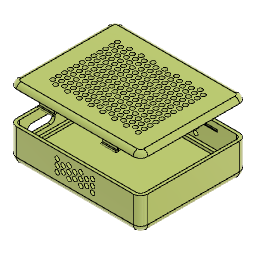
esp32_mesh_node (Autodesk Fusion 360 design; units mm, degrees)
Autodesk Fusion 360 part; units mm, degrees
note: some values were not read from the file. Set by a fixed rule: which sketch regions a step uses.
sketch "Sketch1" plane through (0, 0, 0) normal (0, 0, 1) x (1, 0, 0)
  line L0 (0, 0) -> (44.5, 0)
  line L1 (44.5, 0) -> (44.5, 36)
  line L2 (44.5, 36) -> (0, 36)
  line L3 (0, 36) -> (0, 0)
  dimension "d1" = 44.5
  dimension "d2" = 36
  constraint horizontal L0
  constraint vertical L1
  constraint horizontal L2
  constraint vertical L3
  constraint coincident L0.start L3.end
  measures "d1" distance of L0.start L0.end
  measures "d2" distance of L0.start L2.end
extrude "Extrude1" add sketch "Sketch1" along normal blind 2.5 makes body 1
sketch "Sketch2" plane through (0, 0, 2.5) normal (0, 0, 1) x (-1, 0, 0)
  line L0 (0, -36) -> (0, 0)
  line L1 (0, 0) -> (-44.5, 0)
  line L2 (-44.5, 0) -> (-44.5, -36)
  line L3 (-44.5, -36) -> (0, -36)
  line L4 (-2, -2) -> (-42.5, -2)
  line L5 (-42.5, -2) -> (-42.5, -34)
  line L6 (-42.5, -34) -> (-2, -34)
  line L7 (-2, -34) -> (-2, -2)
  dimension "d5" = -2
extrude "Extrude2" add sketch "Sketch2" along normal blind 8 bodies 1
sketch "Sketch3" plane through (0, 0, 2.5) normal (0, 0, 1) x (-1, 0, 0)
  line L0 (-2, -2) -> (-42.5, -2)
  line L1 (-42.5, -2) -> (-42.5, -34)
  line L2 (-42.5, -34) -> (-2, -34)
  line L3 (-2, -34) -> (-2, -2)
  line L4 (-3.25, -32.75) -> (-41.25, -32.75)
  line L5 (-41.25, -32.75) -> (-41.25, -3.25)
  line L6 (-41.25, -3.25) -> (-3.25, -3.25)
  line L7 (-3.25, -3.25) -> (-3.25, -32.75)
  line L8 (0, -36) -> (0, 0)
  circle A0 centre (-3.25, -32.75) radius 2
  circle A1 centre (-41.25, -32.75) radius 2
  circle A2 centre (-41.25, -3.25) radius 2
  circle A3 centre (-3.25, -3.25) radius 2
  dimension "d18" = 38
  dimension "d20" = 32
  dimension "d21" = 1.25
  dimension "d23" = 40.5
  dimension "d25" = 36
  dimension "d26" = 29.5
  dimension "d27" = 1.25
  dimension "d28" = 4
  dimension "d29" = 4
  dimension "d30" = 4
  dimension "d31" = 4
  constraint horizontal L4
  constraint vertical L5
  constraint horizontal L6
  constraint vertical L7
  constraint coincident L4.start L7.end
  constraint coincident L4.end L5.start
  constraint coincident L5.end L6.start
  constraint coincident L6.end L7.start
  measures "d18" distance of L4.start L4.end
  measures "d20" distance of L0 L2
  measures "d21" distance of L2 L4
  measures "d23" distance of L1 L3
  measures "d25" distance of L8.start L8.end
  measures "d26" distance of L4 L6
  measures "d27" distance of L3 L7
  measures "d28" diameter of A0
  measures "d29" diameter of A1
  measures "d30" diameter of A2
  measures "d31" diameter of A3
extrude "Extrude3" add sketch "Sketch3" along normal blind 1 contours L0 L3 L6 L7 A3 | L0 L1 L5 L6 A2 | L6 L7 A3 | L2 L3 L4 L7 A0 | L5 L6 A2 | L4 L7 A0 | L1 L2 L4 L5 A1 | L4 L5 A1 bodies 1
sketch "Sketch4" plane through (0, 0, 3.5) normal (0, 0, 1) x (-1, 0, 0)
  line L0 (-2, -34) -> (-2, -31.1888)
  arc A0 (-2, -31.1888) -> (-4.8112, -34) centre (-3.25, -32.75) ccw
  line L1 (-4.8112, -34) -> (-2, -34)
  circle A1 centre (-3.25, -32.75) radius 0.9
  line L2 (-2, -2) -> (-4.8112, -2)
  arc A2 (-4.8112, -2) -> (-2, -4.8112) centre (-3.25, -3.25) ccw
  line L3 (-2, -4.8112) -> (-2, -2)
  arc A3 (-42.5, -4.8112) -> (-39.6888, -2) centre (-41.25, -3.25) ccw
  line L4 (-39.6888, -2) -> (-42.5, -2)
  line L5 (-42.5, -2) -> (-42.5, -4.8112)
  arc A4 (-39.6888, -34) -> (-42.5, -31.1888) centre (-41.25, -32.75) ccw
  line L6 (-42.5, -31.1888) -> (-42.5, -34)
  line L7 (-42.5, -34) -> (-39.6888, -34)
  circle A5 centre (-41.25, -32.75) radius 0.9
  circle A6 centre (-41.25, -3.25) radius 0.9
  circle A7 centre (-3.25, -3.25) radius 0.9
  dimension "d34" = 1.8
  dimension "d35" = 1.8
  dimension "d36" = 1.8
  dimension "d37" = 1.8
  constraint concentric A0 A1
  constraint concentric A4 A5
  constraint concentric A3 A6
  constraint concentric A2 A7
  measures "d34" diameter of A1
  measures "d35" diameter of A5
  measures "d36" diameter of A6
  measures "d37" diameter of A7
extrude "Extrude4" add sketch "Sketch4" along normal blind 3 contours A1 | A5 | A6 | A7 bodies 1
sketch "Sketch5" plane through (0, 0, 10.5) normal (0, 0, 1) x (-1, 0, 0)
  line L0 (-2, -2) -> (-2, -34)
  line L1 (-2, -34) -> (-42.5, -34)
  line L2 (-42.5, -34) -> (-42.5, -2)
  line L3 (-42.5, -2) -> (-2, -2)
  line L4 (-44.5, -36) -> (0, -36)
  line L5 (0, -36) -> (0, 0)
  line L6 (0, 0) -> (-44.5, 0)
  line L7 (-44.5, 0) -> (-44.5, -36)
  line L8 (-43.5, -1) -> (-1, -1)
  line L9 (-1, -1) -> (-1, -35)
  line L10 (-1, -35) -> (-43.5, -35)
  line L11 (-43.5, -35) -> (-43.5, -1)
  dimension "d40" = -1
extrude "Extrude5" cut sketch "Sketch5" against normal up to surface (7 mm away) contours L8 L9 L10 L11 bodies 1
sketch "Sketch7" plane through (0, 0, 6.5) normal (0, 0, 1) x (-1, 0, 0)
  circle A0 centre (-3.25, -32.75) radius 1.05
  line L0 (-1, -35) -> (-1, -1)
  line L1 (-1, -1) -> (-43.5, -1)
  line L2 (-43.5, -1) -> (-43.5, -35)
  line L3 (-43.5, -35) -> (-1, -35)
  arc A1 (-42.5, -4.8112) -> (-39.6888, -2) centre (-41.25, -3.25) ccw
  line L4 (-39.6888, -2) -> (-4.8112, -2)
  arc A2 (-4.8112, -2) -> (-2, -4.8112) centre (-3.25, -3.25) ccw
  line L5 (-2, -4.8112) -> (-2, -31.1888)
  arc A3 (-2, -31.1888) -> (-4.8112, -34) centre (-3.25, -32.75) ccw
  line L6 (-4.8112, -34) -> (-39.6888, -34)
  arc A4 (-39.6888, -34) -> (-42.5, -31.1888) centre (-41.25, -32.75) ccw
  line L7 (-42.5, -31.1888) -> (-42.5, -4.8112)
  circle A5 centre (-41.25, -32.75) radius 1.05
  circle A6 centre (-41.25, -3.25) radius 1.05
  circle A7 centre (-3.25, -3.25) radius 1.05
  circle A8 centre (-3.25, -32.75) radius 0.9
  circle A9 centre (-41.25, -32.75) radius 0.9
  circle A10 centre (-41.25, -32.75) radius 0.9
  circle A11 centre (-3.25, -32.75) radius 0.9
  circle A12 centre (-3.25, -3.25) radius 0.9
  circle A13 centre (-41.25, -3.25) radius 0.9
  dimension "d53" = 2.1
  dimension "d54" = 2.1
  dimension "d55" = 2.1
  dimension "d56" = 2.1
  constraint concentric A0 A8
  constraint concentric A5 A9
  constraint concentric A6 A13
  constraint concentric A7 A12
  measures "d53" diameter of A0
  measures "d54" diameter of A5
  measures "d55" diameter of A6
  measures "d56" diameter of A7
extrude "Extrude7" add sketch "Sketch7" against normal blind 1 contours A0 | A5 | A6 | A7 bodies 1
sketch "Sketch8" plane through (0, 0, 6.5) normal (0, 0, 1) x (-1, 0, 0)
  circle A0 centre (-3.25, -32.75) radius 1.05
  line L0 (-1, -35) -> (-1, -1)
  line L1 (-1, -1) -> (-43.5, -1)
  line L2 (-43.5, -1) -> (-43.5, -35)
  line L3 (-43.5, -35) -> (-1, -35)
  arc A1 (-42.5, -4.8112) -> (-39.6888, -2) centre (-41.25, -3.25) ccw
  line L4 (-39.6888, -2) -> (-4.8112, -2)
  arc A2 (-4.8112, -2) -> (-2, -4.8112) centre (-3.25, -3.25) ccw
  line L5 (-2, -4.8112) -> (-2, -31.1888)
  arc A3 (-2, -31.1888) -> (-4.8112, -34) centre (-3.25, -32.75) ccw
  line L6 (-4.8112, -34) -> (-39.6888, -34)
  arc A4 (-39.6888, -34) -> (-42.5, -31.1888) centre (-41.25, -32.75) ccw
  line L7 (-42.5, -31.1888) -> (-42.5, -4.8112)
  line L8 (-3, -31.3622) -> (-3.5, -31.3622)
  line L9 (-3.5, -31.3622) -> (-3.5, -34.2296)
  line L10 (-3.5, -34.2296) -> (-3, -34.2296)
  line L11 (-3, -34.2296) -> (-3, -31.3622)
  line L12 (-41, -31.3358) -> (-41.5, -31.3358)
  line L13 (-41.5, -31.3358) -> (-41.5, -34.1023)
  line L14 (-41.5, -34.1023) -> (-41, -34.1023)
  line L15 (-41, -34.1023) -> (-41, -31.3358)
  line L16 (-41, -1.7959) -> (-41.5, -1.7959)
  line L17 (-41.5, -1.7959) -> (-41.5, -4.5888)
  line L18 (-41.5, -4.5888) -> (-41, -4.5888)
  line L19 (-41, -4.5888) -> (-41, -1.7959)
  line L20 (-3, -1.7959) -> (-3.5, -1.7959)
  line L21 (-3.5, -1.7959) -> (-3.5, -4.5487)
  line L22 (-3.5, -4.5487) -> (-3, -4.5487)
  line L23 (-3, -4.5487) -> (-3, -1.7959)
  circle A5 centre (-41.25, -32.75) radius 0.9
  circle A6 centre (-3.25, -32.75) radius 0.9
  circle A7 centre (-3.25, -3.25) radius 0.9
  circle A8 centre (-41.25, -3.25) radius 0.9
  constraint horizontal L8
  constraint vertical L9
  constraint horizontal L10
  constraint vertical L11
  constraint horizontal L12
  constraint vertical L13
  constraint horizontal L14
  constraint vertical L15
  constraint horizontal L16
  constraint vertical L17
  constraint horizontal L18
  constraint vertical L19
  constraint horizontal L20
  constraint vertical L21
  constraint horizontal L22
  constraint vertical L23
fillet "Fillet3" radius 2.5 4 edges at (0, 0, 5.25) (0, 36, 5.25) (44.5, 36, 5.25) (44.5, 0, 5.25) on bodies 1
fillet "Fillet4" radius 2.5 8 edges at (44.5, 18, 0) (43.7678, 35.2678, 0) (22.25, 36, 0) (0.7322, 35.2678, 0) (0, 18, 0) (0.7322, 0.7322, 0) (22.25, 0, 0) (43.7678, 0.7322, 0) on bodies 1
sketch "Sketch9" plane through (0, 0, 6.5) normal (0, 0, 1) x (-1, 0, 0)
  arc A0 (-42.5, -4.8112) -> (-39.6888, -2) centre (-41.25, -3.25) ccw
  line L0 (-39.6888, -2) -> (-4.8112, -2)
  arc A1 (-4.8112, -2) -> (-2, -4.8112) centre (-3.25, -3.25) ccw
  line L1 (-2, -4.8112) -> (-2, -31.1888)
  arc A2 (-2, -31.1888) -> (-4.8112, -34) centre (-3.25, -32.75) ccw
  line L2 (-4.8112, -34) -> (-39.6888, -34)
  arc A3 (-39.6888, -34) -> (-42.5, -31.1888) centre (-41.25, -32.75) ccw
  line L3 (-42.5, -31.1888) -> (-42.5, -4.8112)
  line L4 (-1, -1) -> (-43.5, -1)
  line L5 (-43.5, -1) -> (-43.5, -35)
  line L6 (-43.5, -35) -> (-1, -35)
  line L7 (-1, -35) -> (-1, -1)
  line L8 (-2.0116, -34.369) -> (-4.4882, -34.369)
  line L9 (-4.4882, -34.369) -> (-4.4882, -33.6146)
  line L10 (-4.4882, -33.6146) -> (-2.0116, -33.6146)
  line L11 (-2.0116, -33.6146) -> (-2.0116, -34.369)
  line L12 (-1.7554, -31.8854) -> (-4.6642, -31.8854)
  line L13 (-4.6642, -31.8854) -> (-4.6642, -31.3358)
  line L14 (-4.6642, -31.3358) -> (-1.7554, -31.3358)
  line L15 (-1.7554, -31.3358) -> (-1.7554, -31.8854)
  line L16 (-40.0537, -34.1608) -> (-42.3788, -34.1608)
  line L17 (-42.3788, -34.1608) -> (-42.3788, -33.6146)
  line L18 (-42.3788, -33.6146) -> (-40.0537, -33.6146)
  line L19 (-40.0537, -33.6146) -> (-40.0537, -34.1608)
  line L20 (-40.0537, -31.8854) -> (-42.5, -31.8854)
  line L21 (-42.5, -31.8854) -> (-42.5, -31.1888)
  line L22 (-42.5, -31.1888) -> (-40.0537, -31.1888)
  line L23 (-40.0537, -31.1888) -> (-40.0537, -31.8854)
  line L24 (-40.0537, -4.1146) -> (-42.1773, -4.1146)
  line L25 (-42.1773, -4.1146) -> (-42.1773, -4.8112)
  line L26 (-42.1773, -4.8112) -> (-40.0537, -4.8112)
  line L27 (-40.0537, -4.8112) -> (-40.0537, -4.1146)
  line L28 (-42.5, -2.3854) -> (-40.0537, -2.3854)
  line L29 (-40.0537, -2.3854) -> (-40.0537, -1.7854)
  line L30 (-40.0537, -1.7854) -> (-42.5, -1.7854)
  line L31 (-42.5, -1.7854) -> (-42.5, -2.3854)
  line L32 (-4.4912, -4.1146) -> (-1.6367, -4.1146)
  line L33 (-1.6367, -4.1146) -> (-1.6367, -5.2006)
  line L34 (-1.6367, -5.2006) -> (-4.4912, -5.2006)
  line L35 (-4.4912, -5.2006) -> (-4.4912, -4.1146)
  line L36 (-2, -2.3854) -> (-5.0179, -2.3854)
  line L37 (-5.0179, -2.3854) -> (-5.0179, -1.7004)
  line L38 (-5.0179, -1.7004) -> (-2, -1.7004)
  line L39 (-2, -1.7004) -> (-2, -2.3854)
  circle A4 centre (-41.25, -32.75) radius 0.9
  circle A5 centre (-3.25, -32.75) radius 0.9
  circle A6 centre (-3.25, -3.25) radius 0.9
  circle A7 centre (-41.25, -3.25) radius 0.9
  circle A8 centre (-3.25, -32.75) radius 1.05
  constraint horizontal L8
  constraint vertical L9
  constraint horizontal L10
  constraint vertical L11
  constraint horizontal L12
  constraint vertical L13
  constraint horizontal L14
  constraint vertical L15
  constraint midpoint A2 L13.end
  constraint horizontal L16
  constraint vertical L17
  constraint horizontal L18
  constraint vertical L19
  constraint horizontal L20
  constraint vertical L21
  constraint horizontal L22
  constraint vertical L23
  constraint coincident A3.end L3.start
  constraint horizontal L24
  constraint vertical L25
  constraint horizontal L26
  constraint vertical L27
  constraint horizontal L28
  constraint vertical L29
  constraint horizontal L30
  constraint vertical L31
  constraint horizontal L32
  constraint vertical L33
  constraint horizontal L34
  constraint vertical L35
  constraint horizontal L36
  constraint vertical L37
  constraint horizontal L38
  constraint vertical L39
sketch "Sketch10" plane through (0, 0, 0) normal (-1, 0, 0) x (0, -1, 0)
  line L0 (-33.5, 2.5) -> (-2.5, 2.5)
  line L1 (-2.5, 2.5) -> (-2.5, 10.5)
  line L2 (-2.5, 10.5) -> (-33.5, 10.5)
  line L3 (-33.5, 10.5) -> (-33.5, 2.5)
  line L4 (-33.65, 3.5) -> (-31.85, 3.5)
  line L5 (-4.15, 3.5) -> (-2.35, 3.5)
  line L6 (-33.65, 3.5) -> (-31.85, 3.5)
  line L7 (-4.15, 3.5) -> (-2.35, 3.5)
  line L8 (-2, 3.5) -> (-5.25, 3.5)
  line L9 (-2, 3.5) -> (-5.25, 3.5)
  line L10 (-4.8112, 3.5) -> (-31.1888, 3.5)
  line L11 (-30.75, 3.5) -> (-34, 3.5)
  line L12 (-30.75, 3.5) -> (-34, 3.5)
  line L13 (-31.1888, 3.5) -> (-4.8112, 3.5)
  line L14 (-1, 3.5) -> (-35, 3.5)
  line L15 (-35, 3.5) -> (-1, 3.5)
  line L16 (-4.15, 5.5) -> (-2.35, 5.5)
  line L17 (-4.15, 3.5) -> (-2.35, 3.5)
  line L18 (-5.3854, 3.5) -> (-14.3254, 3.5)
  line L19 (-14.3254, 3.5) -> (-14.3254, 5.1)
  line L20 (-14.3254, 5.1) -> (-5.3854, 5.1)
  line L21 (-5.3854, 5.1) -> (-5.3854, 3.5)
  line L22 (-14.3254, 5.1) -> (-5.3854, 5.1)
  line L23 (-5.3854, 5.1) -> (-5.3854, 8.26)
  line L24 (-5.3854, 8.26) -> (-14.3254, 8.26)
  line L25 (-14.3254, 8.26) -> (-14.3254, 5.1)
  line L26 (-14.5254, 4.9) -> (-5.1854, 4.9)
  line L27 (-5.1854, 4.9) -> (-5.1854, 8.46)
  line L28 (-5.1854, 8.46) -> (-14.5254, 8.46)
  line L29 (-14.5254, 8.46) -> (-14.5254, 4.9)
  dimension "d73" = 8.94
  dimension "d74" = 1.6
  dimension "d78" = 8.94
  dimension "d79" = 3.16
  dimension "d80" = 0.2
  constraint vertical L19
  constraint horizontal L20
  constraint vertical L21
  constraint coincident L15 L18.start
  constraint horizontal L22
  constraint vertical L23
  constraint horizontal L24
  constraint vertical L25
  measures "d73" distance of L18.start L18.end
  measures "d74" distance of L18.start L20.end
  measures "d78" distance of L19.end L20.end
  measures "d79" distance of L19.end L24.end
extrude "Extrude10" cut sketch "Sketch10" against normal blind 3.85 contours L19 L21 L23 L24 L25 L26 L27 L28 L29 | L19 L20 L21 L22 L26 | L20 L22 L23 L24 L25 bodies 1
fillet "Fillet6" radius 1.435 4 edges at (0.5, 14.5254, 8.46) (0.5, 5.1854, 8.46) (0.5, 5.1854, 4.9) (0.5, 14.5254, 4.9) on bodies 1
fillet "Fillet7" radius 0.5 4 edges at (42.2289, 3.6297, 6.5) (4.2289, 3.6297, 6.5) (42.2289, 33.1297, 6.5) (4.2289, 33.1297, 6.5) on bodies 1
fillet "Fillet8" radius 1.5 4 edges at (1, 1, 7) (1, 35, 7) (43.5, 35, 7) (43.5, 1, 7) on bodies 1
sketch "Sketch11" plane through (0, 0, 10.5) normal (0, 0, 1) x (-1, 0, 0)
  line L0 (-2.5, -35) -> (-42, -35)
  arc A0 (-43.5, -33.5) -> (-42, -35) centre (-42, -33.5) ccw
  line L1 (-43.5, -33.5) -> (-43.5, -2.5)
  arc A1 (-42, -1) -> (-43.5, -2.5) centre (-42, -2.5) ccw
  line L2 (-42, -1) -> (-2.5, -1)
  arc A2 (-1, -2.5) -> (-2.5, -1) centre (-2.5, -2.5) ccw
  line L3 (-1, -2.5) -> (-1, -33.5)
  arc A3 (-2.5, -35) -> (-1, -33.5) centre (-2.5, -33.5) ccw
  arc A4 (-42, 0) -> (-44.5, -2.5) centre (-42, -2.5) ccw
  line L4 (-44.5, -2.5) -> (-44.5, -33.5)
  arc A5 (-44.5, -33.5) -> (-42, -36) centre (-42, -33.5) ccw
  line L5 (-42, -36) -> (-2.5, -36)
  arc A6 (-2.5, -36) -> (0, -33.5) centre (-2.5, -33.5) ccw
  line L6 (0, -33.5) -> (0, -2.5)
  arc A7 (0, -2.5) -> (-2.5, 0) centre (-2.5, -2.5) ccw
  line L7 (-2.5, 0) -> (-42, 0)
extrude "Extrude11" add sketch "Sketch11" along normal blind 1 bodies 1
ref_plane "WorkPlane1" through (0, 0, 15) normal (0, 0, 1) x (1, 0, 0)
sketch "Sketch12" plane through (0, 0, 15) normal (0, 0, 1) x (1, 0, 0)
  arc A0 (43.5, 33.5) -> (42, 35) centre (42, 33.5) ccw
  line L0 (43.5, 33.5) -> (43.5, 2.5)
  arc A1 (42, 1) -> (43.5, 2.5) centre (42, 2.5) ccw
  line L1 (42, 1) -> (2.5, 1)
  arc A2 (1, 2.5) -> (2.5, 1) centre (2.5, 2.5) ccw
  line L2 (1, 2.5) -> (1, 33.5)
  arc A3 (2.5, 35) -> (1, 33.5) centre (2.5, 33.5) ccw
  line L3 (2.5, 35) -> (42, 35)
  line L4 (2.5, 0) -> (42, 0)
  arc A4 (42, 0) -> (44.5, 2.5) centre (42, 2.5) ccw
  line L5 (44.5, 2.5) -> (44.5, 33.5)
  arc A5 (44.5, 33.5) -> (42, 36) centre (42, 33.5) ccw
  line L6 (42, 36) -> (2.5, 36)
  arc A6 (2.5, 36) -> (0, 33.5) centre (2.5, 33.5) ccw
  line L7 (0, 33.5) -> (0, 2.5)
  arc A7 (0, 2.5) -> (2.5, 0) centre (2.5, 2.5) ccw
  arc A8 (42, 1) -> (43.5, 2.5) centre (42, 2.5) ccw
  line L8 (43.5, 2.5) -> (43.5, 33.5)
  arc A9 (43.5, 33.5) -> (42, 35) centre (42, 33.5) ccw
  line L9 (42, 35) -> (2.5, 35)
  arc A10 (2.5, 35) -> (1, 33.5) centre (2.5, 33.5) ccw
  line L10 (1, 33.5) -> (1, 2.5)
  arc A11 (1, 2.5) -> (2.5, 1) centre (2.5, 2.5) ccw
  line L11 (2.5, 1) -> (42, 1)
  arc A12 (42.5, 4.8112) -> (39.6888, 2) centre (41.25, 3.25) ccw
  line L12 (39.6888, 2) -> (4.8112, 2)
  arc A13 (4.8112, 2) -> (2, 4.8112) centre (3.25, 3.25) ccw
  line L13 (2, 4.8112) -> (2, 31.1888)
  arc A14 (2, 31.1888) -> (4.8112, 34) centre (3.25, 32.75) ccw
  line L14 (4.8112, 34) -> (39.6888, 34)
  arc A15 (39.6888, 34) -> (42.5, 31.1888) centre (41.25, 32.75) ccw
  line L15 (42.5, 31.1888) -> (42.5, 4.8112)
  circle A16 centre (41.25, 3.25) radius 0.9
  circle A17 centre (3.25, 3.25) radius 0.9
  circle A18 centre (3.25, 32.75) radius 0.9
  circle A19 centre (41.25, 32.75) radius 0.9
  arc A20 (4.8112, 2) -> (2, 4.8112) centre (3.25, 3.25) ccw
  line L16 (4.8112, 2) -> (39.6888, 2)
  arc A21 (42.5, 4.8112) -> (39.6888, 2) centre (41.25, 3.25) ccw
  line L17 (42.5, 4.8112) -> (42.5, 31.1888)
  arc A22 (39.6888, 34) -> (42.5, 31.1888) centre (41.25, 32.75) ccw
  line L18 (39.6888, 34) -> (4.8112, 34)
  arc A23 (2, 31.1888) -> (4.8112, 34) centre (3.25, 32.75) ccw
  line L19 (2, 31.1888) -> (2, 4.8112)
extrude "Extrude12" add sketch "Sketch12" along normal blind 1.5 separate body contours A0 L0 A1 L1 A2 L2 A3 L3 A8 L8 A9 L9 A10 L10 A11 L11 | L4 A4 L5 A5 L6 A6 L7 A7 | A12 L12 A13 L13 A14 L14 A15 L15 A20 L16 A21 L17 A22 L18 A23 L19 | A16 | A17 | A18 | A19 makes body 2
move_body "Move1" bodies 2 to x (1, 0, 0) y (0, 1, 0) z (0, 0, 1) at (0, 0, 15)
sketch "Sketch13" plane through (0, 0, 30) normal (0, 0, -1) x (1, 0, 0)
  arc A0 (2.5, 0) -> (0, -2.5) centre (2.5, -2.5) ccw
  line L0 (0, -2.5) -> (0, -33.5)
  arc A1 (0, -33.5) -> (2.5, -36) centre (2.5, -33.5) ccw
  line L1 (2.5, -36) -> (42, -36)
  arc A2 (42, -36) -> (44.5, -33.5) centre (42, -33.5) ccw
  line L2 (44.5, -33.5) -> (44.5, -2.5)
  arc A3 (44.5, -2.5) -> (42, 0) centre (42, -2.5) ccw
  line L3 (42, 0) -> (2.5, 0)
  arc A4 (42, -35) -> (43.5, -33.5) centre (42, -33.5) ccw
  line L4 (43.5, -33.5) -> (43.5, -2.5)
  arc A5 (43.5, -2.5) -> (42, -1) centre (42, -2.5) ccw
  line L5 (42, -1) -> (2.5, -1)
  arc A6 (2.5, -1) -> (1, -2.5) centre (2.5, -2.5) ccw
  line L6 (1, -2.5) -> (1, -33.5)
  arc A7 (1, -33.5) -> (2.5, -35) centre (2.5, -33.5) ccw
  line L7 (2.5, -35) -> (42, -35)
  line L8 (2.5, 0) -> (42, 0)
  arc A8 (44.5, -2.5) -> (42, 0) centre (42, -2.5) ccw
  line L9 (44.5, -2.5) -> (44.5, -33.5)
  arc A9 (42, -36) -> (44.5, -33.5) centre (42, -33.5) ccw
  line L10 (42, -36) -> (2.5, -36)
  arc A10 (0, -33.5) -> (2.5, -36) centre (2.5, -33.5) ccw
  line L11 (0, -33.5) -> (0, -2.5)
  arc A11 (2.5, 0) -> (0, -2.5) centre (2.5, -2.5) ccw
  line L12 (9, -1) -> (14, -1)
  line L13 (14, -1) -> (14, -3)
  line L14 (14, -3) -> (9, -3)
  line L15 (9, -3) -> (9, -1)
  line L16 (30.5, -1) -> (35.5, -1)
  line L17 (35.5, -1) -> (35.5, -3)
  line L18 (35.5, -3) -> (30.5, -3)
  line L19 (30.5, -3) -> (30.5, -1)
  line L20 (9, -35) -> (14, -35)
  line L21 (14, -35) -> (14, -33)
  line L22 (14, -33) -> (9, -33)
  line L23 (9, -33) -> (9, -35)
  line L24 (30.5, -35) -> (35.5, -35)
  line L25 (35.5, -35) -> (35.5, -33)
  line L26 (35.5, -33) -> (30.5, -33)
  line L27 (30.5, -33) -> (30.5, -35)
  dimension "d94" = 5
  dimension "d95" = 2
  dimension "d96" = 8
  dimension "d97" = 5
  dimension "d98" = 2
  dimension "d99" = 8
  dimension "d100" = 5
  dimension "d101" = 2
  dimension "d102" = 5
  dimension "d103" = 2
  dimension "d104" = 8
  dimension "d105" = 8
  constraint horizontal L12
  constraint vertical L13
  constraint horizontal L14
  constraint vertical L15
  constraint coincident L5 L12.start
  constraint horizontal L16
  constraint vertical L17
  constraint horizontal L18
  constraint vertical L19
  constraint coincident L5 L16.start
  constraint horizontal L20
  constraint vertical L21
  constraint horizontal L22
  constraint vertical L23
  constraint coincident L7 L20.start
  constraint horizontal L24
  constraint vertical L25
  constraint horizontal L26
  constraint vertical L27
  constraint coincident L7 L24.start
  measures "d94" distance of L12.start L12.end
  measures "d95" distance of L12.start L14.end
  measures "d96" distance of L6 L15
  measures "d97" distance of L16.start L16.end
  measures "d98" distance of L16.start L18.end
  measures "d99" distance of L4 L17
  measures "d100" distance of L20.start L20.end
  measures "d101" distance of L20.start L22.end
  measures "d102" distance of L24.start L24.end
  measures "d103" distance of L24.start L26.end
  measures "d104" distance of L6 L23
  measures "d105" distance of L4 L25
extrude "Extrude13" add sketch "Sketch13" along normal blind 2 contours L7 L24 L25 L26 L27 | L7 L20 L21 L22 L23 | L5 L16 L17 L18 L19 | L5 L12 L13 L14 L15 bodies 2
sketch "Sketch14" plane through (0, 0, 28) normal (0, 0, -1) x (1, 0, 0)
  line L0 (9, -3) -> (14, -3)
  line L1 (14, -3) -> (14, -1)
  line L2 (14, -1) -> (9, -1)
  line L3 (9, -1) -> (9, -3)
  line L4 (9, -3) -> (14, -3)
  line L5 (14, -3) -> (14, -0.5)
  line L6 (14, -0.5) -> (9, -0.5)
  line L7 (9, -0.5) -> (9, -3)
  line L8 (30.5, -3) -> (35.5, -3)
  line L9 (35.5, -3) -> (35.5, -1)
  line L10 (35.5, -1) -> (30.5, -1)
  line L11 (30.5, -1) -> (30.5, -3)
  line L12 (30.5, -33) -> (30.5, -35)
  line L13 (30.5, -35) -> (35.5, -35)
  line L14 (35.5, -35) -> (35.5, -33)
  line L15 (35.5, -33) -> (30.5, -33)
  line L16 (9, -33) -> (9, -35)
  line L17 (9, -35) -> (14, -35)
  line L18 (14, -35) -> (14, -33)
  line L19 (14, -33) -> (9, -33)
  line L20 (30.5, -3) -> (35.5, -3)
  line L21 (35.5, -3) -> (35.5, -0.5)
  line L22 (35.5, -0.5) -> (30.5, -0.5)
  line L23 (30.5, -0.5) -> (30.5, -3)
  line L24 (30.5, -33) -> (35.5, -33)
  line L25 (35.5, -33) -> (35.5, -35.5)
  line L26 (35.5, -35.5) -> (30.5, -35.5)
  line L27 (30.5, -35.5) -> (30.5, -33)
  line L28 (9, -33) -> (14, -33)
  line L29 (14, -33) -> (14, -35.5)
  line L30 (14, -35.5) -> (9, -35.5)
  line L31 (9, -35.5) -> (9, -33)
  dimension "d108" = 2.5
  dimension "d109" = 2.5
  dimension "d110" = 2.5
  dimension "d111" = 2.5
  constraint horizontal L4
  constraint vertical L5
  constraint horizontal L6
  constraint vertical L7
  constraint coincident L0.start L3.end
  constraint horizontal L20
  constraint vertical L21
  constraint horizontal L22
  constraint vertical L23
  constraint coincident L8.start L11.end
  constraint horizontal L24
  constraint vertical L25
  constraint horizontal L26
  constraint vertical L27
  constraint coincident L12.start L15.end
  constraint horizontal L28
  constraint vertical L29
  constraint horizontal L30
  constraint vertical L31
  constraint coincident L16.start L19.end
  measures "d108" distance of L0.start L6.end
  measures "d109" distance of L8.start L22.end
  measures "d110" distance of L12.start L26.end
  measures "d111" distance of L16.start L30.end
extrude "Extrude14" add sketch "Sketch14" along normal blind 0.5 bodies 2
fillet "Fillet9" radius 0.25 4 edges at (33, 35.5, 27.5) (33, 35.5, 28) (11.5, 35.5, 27.5) (11.5, 35.5, 28) on bodies 2
fillet "Fillet10" radius 0.25 4 edges at (33, 0.5, 27.5) (33, 0.5, 28) (11.5, 0.5, 27.5) (11.5, 0.5, 28) on bodies 2
extrude "Extrude15" cut 2 faces at (12.3333, 1, 29.3333) (33.8333, 1, 29.3333) along direction (0, 1, 0) blind 0.2 on bodies 2 bodies 2
extrude "Extrude16" cut 2 faces at (32.1667, 35, 28.6667) (10.6667, 35, 29.3333) along direction (0, -1, 0) blind 0.2 on bodies 2 bodies 2
fillet "Fillet11" radius 1.5 8 edges at (14, 3, 28.75) (9, 3, 28.75) (30.5, 3, 28.75) (35.5, 3, 28.75) (35.5, 33, 28.75) (30.5, 33, 28.75) (14, 33, 28.75) (9, 33, 28.75) on bodies 2
fillet "Fillet12" radius 1 20 edges at (30.5, 34.65, 30) (30.9393, 33.4393, 30) (33, 33, 30) (35.0607, 33.4393, 30) (35.5, 34.65, 30) (9, 34.65, 30) (9.4393, 33.4393, 30) (11.5, 33, 30) (13.5607, 33.4393, 30) (14, 34.65, 30) (30.5, 1.35, 30) (30.9393, 2.5607, 30) (33, 3, 30) (35.0607, 2.5607, 30) (35.5, 1.35, 30) (14, 1.35, 30) (13.5607, 2.5607, 30) (11.5, 3, 30) (9.4393, 2.5607, 30) (9, 1.35, 30) on bodies 2
ref_plane "WorkPlane2" through (11.5, 2, 9.5) normal (0, 0, 1) x (-1, 0, 0)
sketch "Sketch17" plane through (11.5, 2, 9.5) normal (0, 0, 1) x (1, 0, 0)
  arc A0 (-1, 1) -> (-2.5, -0.5) centre (-1, -0.5) ccw
  line L0 (-1, 1) -> (1, 1)
  arc A1 (2.5, -0.5) -> (1, 1) centre (1, -0.5) ccw
  line L1 (2.5, -0.5) -> (2.5, -1.25)
  line L2 (2.5, -1.25) -> (-2.5, -1.25)
  line L3 (-2.5, -1.25) -> (-2.5, -0.5)
  line L4 (-2.5, -1.5) -> (-2.5, -1.25)
  line L5 (-2.5, -1.25) -> (2.5, -1.25)
  line L6 (2.5, -1.25) -> (2.5, -1.5)
  line L7 (2.5, -1.25) -> (-2.5, -1.25)
  arc A2 (24, -0.5) -> (22.5, 1) centre (22.5, -0.5) ccw
  line L8 (24, -0.5) -> (24, -1.25)
  line L9 (24, -1.25) -> (19, -1.25)
  line L10 (19, -1.25) -> (19, -0.5)
  arc A3 (20.5, 1) -> (19, -0.5) centre (20.5, -0.5) ccw
  line L11 (20.5, 1) -> (22.5, 1)
  line L12 (19, -1.5) -> (19, -1.25)
  line L13 (19, -1.25) -> (24, -1.25)
  line L14 (24, -1.25) -> (24, -1.5)
  line L15 (24, -1.25) -> (19, -1.25)
  line L16 (2.5, 33.25) -> (-2.5, 33.25)
  arc A4 (-2.5, 32.5) -> (-1, 31) centre (-1, 32.5) ccw
  line L17 (-2.5, 32.5) -> (-2.5, 33.25)
  line L18 (-2.5, 33.25) -> (2.5, 33.25)
  line L19 (2.5, 33.25) -> (2.5, 32.5)
  arc A5 (1, 31) -> (2.5, 32.5) centre (1, 32.5) ccw
  line L20 (1, 31) -> (-1, 31)
  arc A6 (19, 32.5) -> (20.5, 31) centre (20.5, 32.5) ccw
  line L21 (19, 32.5) -> (19, 33.25)
  line L22 (19, 33.25) -> (24, 33.25)
  line L23 (24, 33.25) -> (24, 32.5)
  arc A7 (22.5, 31) -> (24, 32.5) centre (22.5, 32.5) ccw
  line L24 (22.5, 31) -> (20.5, 31)
  line L25 (24, 33.5) -> (24, 33.25)
  line L26 (24, 33.25) -> (19, 33.25)
  line L27 (19, 33.25) -> (19, 33.5)
  line L28 (19, 33.25) -> (24, 33.25)
  line L29 (2.6, 33.35) -> (2.6, 32.5)
  arc A8 (1, 30.9) -> (2.6, 32.5) centre (1, 32.5) ccw
  line L30 (1, 30.9) -> (-1, 30.9)
  arc A9 (-2.6, 32.5) -> (-1, 30.9) centre (-1, 32.5) ccw
  line L31 (-2.6, 32.5) -> (-2.6, 33.35)
  line L32 (-2.6, 33.35) -> (2.6, 33.35)
  line L33 (22.5, 30.9) -> (20.5, 30.9)
  arc A10 (18.9, 32.5) -> (20.5, 30.9) centre (20.5, 32.5) ccw
  line L34 (18.9, 32.5) -> (18.9, 33.35)
  line L35 (18.9, 33.35) -> (24.1, 33.35)
  line L36 (24.1, 33.35) -> (24.1, 32.5)
  arc A11 (22.5, 30.9) -> (24.1, 32.5) centre (22.5, 32.5) ccw
  line L37 (20.5, 1.1) -> (22.5, 1.1)
  arc A12 (24.1, -0.5) -> (22.5, 1.1) centre (22.5, -0.5) ccw
  line L38 (24.1, -0.5) -> (24.1, -1.35)
  line L39 (24.1, -1.35) -> (18.9, -1.35)
  line L40 (18.9, -1.35) -> (18.9, -0.5)
  arc A13 (20.5, 1.1) -> (18.9, -0.5) centre (20.5, -0.5) ccw
  line L41 (-1, 1.1) -> (1, 1.1)
  arc A14 (2.6, -0.5) -> (1, 1.1) centre (1, -0.5) ccw
  line L42 (2.6, -0.5) -> (2.6, -1.35)
  line L43 (2.6, -1.35) -> (-2.6, -1.35)
  line L44 (-2.6, -1.35) -> (-2.6, -0.5)
  arc A15 (-1, 1.1) -> (-2.6, -0.5) centre (-1, -0.5) ccw
  dimension "d131" = 0.1
  dimension "d132" = 0.1
  dimension "d133" = 0.1
  dimension "d134" = 0.1
extrude "Extrude17" cut sketch "Sketch17" along normal blind 0.1 and the other way blind 0.6 contours A0 L0 A1 L1 L2 L3 L5 L7 | A2 L8 L9 L10 A3 L11 L13 L15 | L16 A4 L17 L18 L19 A5 L20 | A6 L21 L22 L23 A7 L24 L26 L28 bodies 1
move_body "Move2" bodies 2 to x (1, 0, 0) y (0, 1, 0) z (0, 0, 1) at (0, 0, -18.5)
fillet "Fillet13" radius 1.5 8 edges at (22.25, 0, 13) (43.7678, 0.7322, 13) (44.5, 18, 13) (43.7678, 35.2678, 13) (22.25, 36, 13) (0.7322, 35.2678, 13) (0, 18, 13) (0.7322, 0.7322, 13) on bodies 2
move_body "Move3" bodies 2 to x (1, 0, 0) y (0, 1, 0) z (0, 0, 1) at (0, 0, 35)
sketch "Sketch18" plane through (0, 0, 0) normal (0, -1, 0) x (1, 0, 0)
  line L0 (2.5, 2.5) -> (42, 2.5)
  line L1 (42, 2.5) -> (42, 11.5)
  line L2 (42, 11.5) -> (2.5, 11.5)
  line L3 (2.5, 11.5) -> (2.5, 2.5)
  circle A0 centre (16.25, 9) radius 0.75
  circle A1 centre (16.25, 7) radius 0.75
  circle A2 centre (16.25, 5) radius 0.75
  circle A3 centre (18.25, 8) radius 0.75
  circle A4 centre (18.25, 6) radius 0.75
  circle A5 centre (20.25, 9) radius 0.75
  circle A6 centre (20.25, 7) radius 0.75
  circle A7 centre (20.25, 5) radius 0.75
  circle A8 centre (22.25, 6) radius 0.75
  circle A9 centre (22.25, 8) radius 0.75
  circle A10 centre (24.25, 9) radius 0.75
  circle A11 centre (24.25, 7) radius 0.75
  circle A12 centre (24.25, 5) radius 0.75
  circle A13 centre (26.25, 6) radius 0.75
  circle A14 centre (26.25, 8) radius 0.75
  circle A15 centre (28.25, 9) radius 0.75
  circle A16 centre (28.25, 7) radius 0.75
  circle A17 centre (28.25, 5) radius 0.75
  dimension "d141" = 1.5
  dimension "d142" = 2.5
  dimension "d143" = 13.75
  dimension "d144" = 1.5
  dimension "d145" = 2
  dimension "d146" = 1.5
  dimension "d147" = 2
  dimension "d148" = 2.5
  dimension "d149" = 1.5
  dimension "d150" = 1
  dimension "d151" = 2
  dimension "d152" = 1.5
  dimension "d153" = 2
  dimension "d154" = 1
  dimension "d157" = 4
  dimension "d158" = 0
  dimension "d159" = 13.75
  measures "d141" diameter of A0
  measures "d142" distance of L2 A0.centre
  measures "d143" distance of L3 A0.centre
  measures "d144" diameter of A1
  measures "d145" distance of A0.centre A1.centre
  measures "d146" diameter of A2
  measures "d147" distance of A1.centre A2.centre
  measures "d148" distance of L0 A2.centre
  measures "d149" diameter of A3
  measures "d150" vertical distance of A0.centre A3.centre
  measures "d151" horizontal distance of A0.centre A3.centre
  measures "d152" diameter of A4
  measures "d153" horizontal distance of A1.centre A4.centre
  measures "d154" vertical distance of A2.centre A4.centre
  measures "d159" distance of L1 A15.centre
extrude "Extrude18" cut sketch "Sketch18" against normal blind 52 contours A0 | A1 | A2 | A3 | A4 | A5 | A6 | A7 | A8 | A9 | A10 | A11 | A12 | A13 | A14 | A15 | A16 | A17 bodies 1
sketch "Sketch19" plane through (0, 0, 48) normal (0, 0, 1) x (-1, 0, 0)
  line L0 (-2.5, -1.5) -> (-42, -1.5)
  arc A0 (-42, -1.5) -> (-43, -2.5) centre (-42, -2.5) ccw
  line L1 (-43, -2.5) -> (-43, -33.5)
  arc A1 (-43, -33.5) -> (-42, -34.5) centre (-42, -33.5) ccw
  line L2 (-42, -34.5) -> (-2.5, -34.5)
  arc A2 (-2.5, -34.5) -> (-1.5, -33.5) centre (-2.5, -33.5) ccw
  line L3 (-1.5, -33.5) -> (-1.5, -2.5)
  arc A3 (-1.5, -2.5) -> (-2.5, -1.5) centre (-2.5, -2.5) ccw
  circle A4 centre (-7.25, -29.5) radius 0.75
  arc A5 (-30.5, -34.5) -> (-32, -33) centre (-32, -34.5) ccw
  line L4 (-30.5, -34.5) -> (-30.5, -35.25)
  line L5 (-30.5, -35.25) -> (-35.5, -35.25)
  line L6 (-35.5, -35.25) -> (-35.5, -34.5)
  arc A6 (-34, -33) -> (-35.5, -34.5) centre (-34, -34.5) ccw
  line L7 (-34, -33) -> (-32, -33)
  arc A7 (-9, -34.5) -> (-10.5, -33) centre (-10.5, -34.5) ccw
  line L8 (-9, -34.5) -> (-9, -35.25)
  line L9 (-9, -35.25) -> (-14, -35.25)
  line L10 (-14, -35.25) -> (-14, -34.5)
  arc A8 (-12.5, -33) -> (-14, -34.5) centre (-12.5, -34.5) ccw
  line L11 (-12.5, -33) -> (-10.5, -33)
  line L12 (-10.5, -32) -> (-10.5, -33)
  arc A9 (-8, -34.5) -> (-10.5, -32) centre (-10.5, -34.5) ccw
  line L13 (-8, -34.5) -> (-9, -34.5)
  arc A10 (-9, -34.5) -> (-10.5, -33) centre (-10.5, -34.5) ccw
  line L14 (-12.5, -32) -> (-12.5, -33)
  line L15 (-12.5, -32) -> (-10.5, -32)
  line L16 (-10.5, -32) -> (-10.5, -33)
  line L17 (-10.5, -33) -> (-12.5, -33)
  line L18 (-15, -34.5) -> (-14, -34.5)
  arc A11 (-12.5, -32) -> (-15, -34.5) centre (-12.5, -34.5) ccw
  line L19 (-12.5, -32) -> (-12.5, -33)
  arc A12 (-12.5, -33) -> (-14, -34.5) centre (-12.5, -34.5) ccw
  arc A13 (-10.5, -3) -> (-9, -1.5) centre (-10.5, -1.5) ccw
  line L20 (-10.5, -3) -> (-12.5, -3)
  arc A14 (-14, -1.5) -> (-12.5, -3) centre (-12.5, -1.5) ccw
  line L21 (-14, -1.5) -> (-14, -0.75)
  line L22 (-14, -0.75) -> (-9, -0.75)
  line L23 (-9, -0.75) -> (-9, -1.5)
  arc A15 (-35.5, -1.5) -> (-34, -3) centre (-34, -1.5) ccw
  line L24 (-35.5, -1.5) -> (-35.5, -0.75)
  line L25 (-35.5, -0.75) -> (-30.5, -0.75)
  line L26 (-30.5, -0.75) -> (-30.5, -1.5)
  arc A16 (-32, -3) -> (-30.5, -1.5) centre (-32, -1.5) ccw
  line L27 (-32, -3) -> (-34, -3)
  line L28 (-29.5, -1.5) -> (-30.5, -1.5)
  arc A17 (-32, -4) -> (-29.5, -1.5) centre (-32, -1.5) ccw
  line L29 (-32, -4) -> (-32, -3)
  arc A18 (-32, -3) -> (-30.5, -1.5) centre (-32, -1.5) ccw
  line L30 (-32, -4) -> (-32, -3)
  line L31 (-32, -4) -> (-34, -4)
  line L32 (-34, -4) -> (-34, -3)
  line L33 (-34, -3) -> (-32, -3)
  arc A19 (-36.5, -1.5) -> (-34, -4) centre (-34, -1.5) ccw
  line L34 (-32, -32) -> (-32, -33)
  arc A20 (-29.5, -34.5) -> (-32, -32) centre (-32, -34.5) ccw
  line L35 (-29.5, -34.5) -> (-30.5, -34.5)
  arc A21 (-30.5, -34.5) -> (-32, -33) centre (-32, -34.5) ccw
  line L36 (-34, -32) -> (-34, -33)
  line L37 (-34, -32) -> (-32, -32)
  line L38 (-32, -32) -> (-32, -33)
  line L39 (-32, -33) -> (-34, -33)
  line L40 (-10.5, -4) -> (-10.5, -3)
  line L41 (-10.5, -4) -> (-12.5, -4)
  line L42 (-12.5, -4) -> (-12.5, -3)
  line L43 (-12.5, -3) -> (-10.5, -3)
  line L44 (-8, -1.5) -> (-9, -1.5)
  arc A22 (-10.5, -4) -> (-8, -1.5) centre (-10.5, -1.5) ccw
  line L45 (-10.5, -4) -> (-10.5, -3)
  arc A23 (-10.5, -3) -> (-9, -1.5) centre (-10.5, -1.5) ccw
  circle A24 centre (-7.25, -27.5) radius 0.75
  circle A25 centre (-9.25, -28.5) radius 0.75
  circle A26 centre (-9.25, -26.5) radius 0.75
  circle A27 centre (-11.25, -29.5) radius 0.75
  circle A28 centre (-11.25, -27.5) radius 0.75
  circle A29 centre (-13.25, -26.5) radius 0.75
  circle A30 centre (-13.25, -28.5) radius 0.75
  circle A31 centre (-15.25, -29.5) radius 0.75
  circle A32 centre (-15.25, -27.5) radius 0.75
  circle A33 centre (-17.25, -26.5) radius 0.75
  circle A34 centre (-17.25, -28.5) radius 0.75
  circle A35 centre (-19.25, -29.5) radius 0.75
  circle A36 centre (-19.25, -27.5) radius 0.75
  circle A37 centre (-21.25, -26.5) radius 0.75
  circle A38 centre (-21.25, -28.5) radius 0.75
  circle A39 centre (-23.25, -29.5) radius 0.75
  circle A40 centre (-23.25, -27.5) radius 0.75
  circle A41 centre (-25.25, -26.5) radius 0.75
  circle A42 centre (-25.25, -28.5) radius 0.75
  circle A43 centre (-27.25, -29.5) radius 0.75
  circle A44 centre (-27.25, -27.5) radius 0.75
  circle A45 centre (-29.25, -26.5) radius 0.75
  circle A46 centre (-29.25, -28.5) radius 0.75
  circle A47 centre (-31.25, -29.5) radius 0.75
  circle A48 centre (-31.25, -27.5) radius 0.75
  circle A49 centre (-33.25, -26.5) radius 0.75
  circle A50 centre (-33.25, -28.5) radius 0.75
  circle A51 centre (-35.25, -29.5) radius 0.75
  circle A52 centre (-35.25, -27.5) radius 0.75
  circle A53 centre (-37.25, -26.5) radius 0.75
  circle A54 centre (-37.25, -28.5) radius 0.75
  circle A55 centre (-7.25, -25.5) radius 0.75
  circle A56 centre (-7.25, -23.5) radius 0.75
  circle A57 centre (-9.25, -22.5) radius 0.75
  circle A58 centre (-9.25, -24.5) radius 0.75
  circle A59 centre (-11.25, -25.5) radius 0.75
  circle A60 centre (-11.25, -23.5) radius 0.75
  circle A61 centre (-13.25, -22.5) radius 0.75
  circle A62 centre (-13.25, -24.5) radius 0.75
  circle A63 centre (-15.25, -25.5) radius 0.75
  circle A64 centre (-15.25, -23.5) radius 0.75
  circle A65 centre (-17.25, -22.5) radius 0.75
  circle A66 centre (-17.25, -24.5) radius 0.75
  circle A67 centre (-19.25, -25.5) radius 0.75
  circle A68 centre (-19.25, -23.5) radius 0.75
  circle A69 centre (-21.25, -22.5) radius 0.75
  circle A70 centre (-21.25, -24.5) radius 0.75
  circle A71 centre (-23.25, -25.5) radius 0.75
  circle A72 centre (-23.25, -23.5) radius 0.75
  circle A73 centre (-25.25, -22.5) radius 0.75
  circle A74 centre (-25.25, -24.5) radius 0.75
  circle A75 centre (-27.25, -25.5) radius 0.75
  circle A76 centre (-27.25, -23.5) radius 0.75
  circle A77 centre (-29.25, -22.5) radius 0.75
  circle A78 centre (-29.25, -24.5) radius 0.75
  circle A79 centre (-31.25, -25.5) radius 0.75
  circle A80 centre (-31.25, -23.5) radius 0.75
  circle A81 centre (-33.25, -22.5) radius 0.75
  circle A82 centre (-33.25, -24.5) radius 0.75
  circle A83 centre (-35.25, -25.5) radius 0.75
  circle A84 centre (-35.25, -23.5) radius 0.75
  circle A85 centre (-37.25, -22.5) radius 0.75
  circle A86 centre (-37.25, -24.5) radius 0.75
  circle A87 centre (-7.25, -21.5) radius 0.75
  circle A88 centre (-7.25, -19.5) radius 0.75
  circle A89 centre (-9.25, -18.5) radius 0.75
  circle A90 centre (-9.25, -20.5) radius 0.75
  circle A91 centre (-11.25, -21.5) radius 0.75
  circle A92 centre (-11.25, -19.5) radius 0.75
  circle A93 centre (-13.25, -18.5) radius 0.75
  circle A94 centre (-13.25, -20.5) radius 0.75
  circle A95 centre (-15.25, -21.5) radius 0.75
  circle A96 centre (-15.25, -19.5) radius 0.75
  circle A97 centre (-17.25, -18.5) radius 0.75
  circle A98 centre (-17.25, -20.5) radius 0.75
  circle A99 centre (-19.25, -21.5) radius 0.75
  circle A100 centre (-19.25, -19.5) radius 0.75
  circle A101 centre (-21.25, -18.5) radius 0.75
  circle A102 centre (-21.25, -20.5) radius 0.75
  circle A103 centre (-23.25, -21.5) radius 0.75
  circle A104 centre (-23.25, -19.5) radius 0.75
  circle A105 centre (-25.25, -18.5) radius 0.75
  circle A106 centre (-25.25, -20.5) radius 0.75
  circle A107 centre (-27.25, -21.5) radius 0.75
  circle A108 centre (-27.25, -19.5) radius 0.75
  circle A109 centre (-29.25, -18.5) radius 0.75
  circle A110 centre (-29.25, -20.5) radius 0.75
  circle A111 centre (-31.25, -21.5) radius 0.75
  circle A112 centre (-31.25, -19.5) radius 0.75
  circle A113 centre (-33.25, -18.5) radius 0.75
  circle A114 centre (-33.25, -20.5) radius 0.75
  circle A115 centre (-35.25, -21.5) radius 0.75
  circle A116 centre (-35.25, -19.5) radius 0.75
  circle A117 centre (-37.25, -18.5) radius 0.75
  circle A118 centre (-37.25, -20.5) radius 0.75
  circle A119 centre (-7.25, -17.5) radius 0.75
  circle A120 centre (-7.25, -15.5) radius 0.75
  circle A121 centre (-9.25, -14.5) radius 0.75
  circle A122 centre (-9.25, -16.5) radius 0.75
  circle A123 centre (-11.25, -17.5) radius 0.75
  circle A124 centre (-11.25, -15.5) radius 0.75
  circle A125 centre (-13.25, -14.5) radius 0.75
  circle A126 centre (-13.25, -16.5) radius 0.75
  circle A127 centre (-15.25, -17.5) radius 0.75
  circle A128 centre (-15.25, -15.5) radius 0.75
  circle A129 centre (-17.25, -14.5) radius 0.75
  circle A130 centre (-17.25, -16.5) radius 0.75
  circle A131 centre (-19.25, -17.5) radius 0.75
  circle A132 centre (-19.25, -15.5) radius 0.75
  circle A133 centre (-21.25, -14.5) radius 0.75
  circle A134 centre (-21.25, -16.5) radius 0.75
  circle A135 centre (-23.25, -17.5) radius 0.75
  circle A136 centre (-23.25, -15.5) radius 0.75
  circle A137 centre (-25.25, -14.5) radius 0.75
  circle A138 centre (-25.25, -16.5) radius 0.75
  circle A139 centre (-27.25, -17.5) radius 0.75
  circle A140 centre (-27.25, -15.5) radius 0.75
  circle A141 centre (-29.25, -14.5) radius 0.75
  circle A142 centre (-29.25, -16.5) radius 0.75
  circle A143 centre (-31.25, -17.5) radius 0.75
  circle A144 centre (-31.25, -15.5) radius 0.75
  circle A145 centre (-33.25, -14.5) radius 0.75
  circle A146 centre (-33.25, -16.5) radius 0.75
  circle A147 centre (-35.25, -17.5) radius 0.75
  circle A148 centre (-35.25, -15.5) radius 0.75
  circle A149 centre (-37.25, -14.5) radius 0.75
  circle A150 centre (-37.25, -16.5) radius 0.75
  circle A151 centre (-7.25, -13.5) radius 0.75
  circle A152 centre (-7.25, -11.5) radius 0.75
  circle A153 centre (-9.25, -10.5) radius 0.75
  circle A154 centre (-9.25, -12.5) radius 0.75
  circle A155 centre (-11.25, -13.5) radius 0.75
  circle A156 centre (-11.25, -11.5) radius 0.75
  circle A157 centre (-13.25, -10.5) radius 0.75
  circle A158 centre (-13.25, -12.5) radius 0.75
  circle A159 centre (-15.25, -13.5) radius 0.75
  circle A160 centre (-15.25, -11.5) radius 0.75
  circle A161 centre (-17.25, -10.5) radius 0.75
  circle A162 centre (-17.25, -12.5) radius 0.75
  circle A163 centre (-19.25, -13.5) radius 0.75
  circle A164 centre (-19.25, -11.5) radius 0.75
  circle A165 centre (-21.25, -10.5) radius 0.75
  circle A166 centre (-21.25, -12.5) radius 0.75
  circle A167 centre (-23.25, -13.5) radius 0.75
  circle A168 centre (-23.25, -11.5) radius 0.75
  circle A169 centre (-25.25, -10.5) radius 0.75
  circle A170 centre (-25.25, -12.5) radius 0.75
  circle A171 centre (-27.25, -13.5) radius 0.75
  circle A172 centre (-27.25, -11.5) radius 0.75
  circle A173 centre (-29.25, -10.5) radius 0.75
  circle A174 centre (-29.25, -12.5) radius 0.75
  circle A175 centre (-31.25, -13.5) radius 0.75
  circle A176 centre (-31.25, -11.5) radius 0.75
  circle A177 centre (-33.25, -10.5) radius 0.75
  circle A178 centre (-33.25, -12.5) radius 0.75
  circle A179 centre (-35.25, -13.5) radius 0.75
  circle A180 centre (-35.25, -11.5) radius 0.75
  circle A181 centre (-37.25, -10.5) radius 0.75
  circle A182 centre (-37.25, -12.5) radius 0.75
  circle A183 centre (-7.25, -9.5) radius 0.75
  circle A184 centre (-7.25, -7.5) radius 0.75
  circle A185 centre (-9.25, -6.5) radius 0.75
  circle A186 centre (-9.25, -8.5) radius 0.75
  circle A187 centre (-11.25, -9.5) radius 0.75
  circle A188 centre (-11.25, -7.5) radius 0.75
  circle A189 centre (-13.25, -6.5) radius 0.75
  circle A190 centre (-13.25, -8.5) radius 0.75
  circle A191 centre (-15.25, -9.5) radius 0.75
  circle A192 centre (-15.25, -7.5) radius 0.75
  circle A193 centre (-17.25, -6.5) radius 0.75
  circle A194 centre (-17.25, -8.5) radius 0.75
  circle A195 centre (-19.25, -9.5) radius 0.75
  circle A196 centre (-19.25, -7.5) radius 0.75
  circle A197 centre (-21.25, -6.5) radius 0.75
  circle A198 centre (-21.25, -8.5) radius 0.75
  circle A199 centre (-23.25, -9.5) radius 0.75
  circle A200 centre (-23.25, -7.5) radius 0.75
  circle A201 centre (-25.25, -6.5) radius 0.75
  circle A202 centre (-25.25, -8.5) radius 0.75
  circle A203 centre (-27.25, -9.5) radius 0.75
  circle A204 centre (-27.25, -7.5) radius 0.75
  circle A205 centre (-29.25, -6.5) radius 0.75
  circle A206 centre (-29.25, -8.5) radius 0.75
  circle A207 centre (-31.25, -9.5) radius 0.75
  circle A208 centre (-31.25, -7.5) radius 0.75
  circle A209 centre (-33.25, -6.5) radius 0.75
  circle A210 centre (-33.25, -8.5) radius 0.75
  circle A211 centre (-35.25, -9.5) radius 0.75
  circle A212 centre (-35.25, -7.5) radius 0.75
  circle A213 centre (-37.25, -6.5) radius 0.75
  circle A214 centre (-37.25, -8.5) radius 0.75
  point P0 (-10.5, -32)
  point P1 (-34, -3)
  point P2 (-32, -32)
  point P3 (-34, -32)
  dimension "d162" = 1.5
  dimension "d163" = 5
  dimension "d164" = 5.75
  dimension "d165" = 1.5
  dimension "d166" = 2
  dimension "d167" = 1.5
  dimension "d168" = 2
  dimension "d169" = 1
  dimension "d170" = 1.5
  dimension "d171" = 2
  dimension "d172" = 2
  dimension "d175" = -4
  dimension "d176" = 4
  measures "d162" diameter of A4
  measures "d163" distance of L2 A4.centre
  measures "d164" distance of L3 A4.centre
  measures "d165" diameter of A24
  measures "d166" distance of A4.centre A24.centre
  measures "d167" diameter of A25
  measures "d168" horizontal distance of A4.centre A25.centre
  measures "d169" vertical distance of A4.centre A25.centre
  measures "d170" diameter of A26
  measures "d171" distance of A25.centre A26.centre
  measures "d172" horizontal distance of A24.centre A26.centre
extrude "Extrude19" cut sketch "Sketch19" against normal blind 9 contours A4 | A24 | A25 | A26 | A27 | A28 | A29 | A30 | A31 | A32 | A33 | A34 | A35 | A36 | A37 | A38 | A39 | A40 | A41 | A42 | A43 | A44 | A45 | A46 | A47 | A48 | A49 | A50 | A51 | A52 | A53 | A54 | A55 | A56 | A57 | A58 | A59 | A60 | A61 | A62 | A63 | A64 | A65 | A66 | A67 | A68 | A69 | A70 | A71 | A72 | A73 | A74 | A75 | A76 | A77 | A78 | A79 | A80 | A81 | A82 | A83 | A84 | A85 | A86 | A87 | A88 | A89 | A90 | A91 | A92 | A93 | A94 | A95 | A96 | A97 | A98 | A99 | A100 | A101 | A102 | A103 | A104 | A105 | A106 | A107 | A108 | A109 | A110 | A111 | A112 | A113 | A114 | A115 | A116 | A117 | A118 | A119 | A120 | A121 | A122 | A123 | A124 | A125 | A126 | A127 | A128 | A129 | A130 | A131 | A132 | A133 | A134 | A135 | A136 | A137 | A138 | A139 | A140 | A141 | A142 | A143 | A144 | A145 | A146 | A147 | A148 | A149 | A150 | A151 | A152 | A153 | A154 | A155 | A156 | A157 | A158 | A159 | A160 | A161 | A162 | A163 | A164 | A165 | A166 | A167 | A168 | A169 | A170 | A171 | A172 | A173 | A174 | A175 | A176 | A177 | A178 | A179 | A180 | A181 | A182 | A183 | A184 | A185 | A186 | A187 | A188 | A189 | A190 | A191 | A192 | A193 | A194 | A195 | A196 | A197 | A198 | A199 | A200 | A201 | A202 | A203 | A204 | A205 | A206 | A207 | A208 | A209 | A210 | A211 | A212 | A213 | A214 bodies 2
move_body "Move4" bodies 2 to x (1, 0, 0) y (0, 1, 0) z (0, 0, 1) at (0, 0, -24)
equation "d21 = ( d20 - d26 ) / 2"
equation "d27 = ( d23 - d18 ) / 2"
